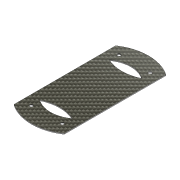
# Autodesk Inventor part: plyta_odbiornik
Saved by Autodesk Inventor 2017 (Build 210142000, 142)
## iProperties
Created: 2017-05-11
Part Number: plyta_odbiornik
Material: Ogólny
Document SubType Name: Modeling
Designer: Kuba01
Density: 1 g/cm^3
Appearance: Domyślna
Author: Kuba01
Autodesk Inventor part; units mm, degrees
ref_plane "YZ Plane" through (0, 0, 0) normal (1, 0, 0) x (0, 1, 0)
ref_plane "XZ Plane" through (0, 0, 0) normal (0, 1, 0) x (-1, 0, 0)
ref_plane "XY Plane" through (0, 0, 0) normal (0, 0, 1) x (1, 0, 0)
sketch "Szkic1" plane through (0, 0, 0) normal (0, 0, 1) x (1, 0, 0)
  circle A0 centre (-19, 53.736463) radius 2
  line L0 (0, -102.826606) -> (0, 109.459635)
  circle A1 centre (51.489502, -156.180896) radius 2
  circle A2 centre (-19, -53.736463) radius 2
  circle A3 centre (19, -53.736463) radius 2
  spline S0 degree 3 poles (-19.948357, 42.291714) (-7.484612, 36.499399) (6.838806, 36.499399) (19.884685, 42.334177) knots -2 -2 -2 -2 -1 -1 -1 -1
  spline S1 degree 3 poles (19.884685, 42.334177) (18.683547, 43.134298) (16.314211, 44.578944) (13.440795, 46.011363) (10.633281, 47.178527) (8.438356, 47.906787) (5.748573, 48.576507) (3.633449, 48.926153) (1.014806, 49.141741) (-1.070138, 49.1397) (-3.689231, 48.918937) (-5.805048, 48.565032) (-8.496008, 47.889736) (-10.692066, 47.156791) (-13.501106, 45.983476) (-16.376096, 44.544624) (-18.746641, 43.094581) (-19.948357, 42.291714) knots -1.92878405 -1.92878405 -1.92878405 -1.92878405 -1.85742515 -1.78606626 -1.75038681 -1.67902792 -1.64334847 -1.57198957 -1.53631013 -1.46495123 -1.42927178 -1.35791289 -1.32223344 -1.25087454 -1.2151951 -1.1438362 -1.0724773 -1.0724773 -1.0724773 -1.0724773
  spline S2 degree 3 poles (-19.948357, -42.291714) (-7.484612, -36.499399) (6.838806, -36.499399) (19.884685, -42.334177) (19.887771, -42.335557) (19.890857, -42.336938) (19.893943, -42.338318) knots -2 -2 -2 -2 -1 -1 -1 -0.99976344 -0.99976344 -0.99976344 -0.99976344
  arc A4 (10.816477, 63.441394) -> (10.816477, 63.441394) centre (0.029646, 15.697095) ccw
  line L1 (-30.717431, -63.122795) -> (-30.717431, 61.299929)
  line L2 (30.776723, 61.29993) -> (30.717431, -63.122795)
  arc A5 (46.460279, 45.179229) -> (46.388819, 45.291469) centre (0.029646, 15.697095) ccw
  arc A6 (30.776723, 61.29993) -> (-30.717431, 61.299929) centre (0.029646, 15.697095) ccw
  arc A7 (-30.717431, -63.122795) -> (30.717431, -63.122795) centre (0, -17.5) ccw
  spline S3 degree 3 poles (19.884685, -42.334177) (18.683547, -43.134298) (16.314211, -44.578944) (13.440795, -46.011363) (10.633281, -47.178527) (8.438356, -47.906787) (5.748573, -48.576507) (3.633449, -48.926153) (1.014806, -49.141741) (-1.070138, -49.1397) (-3.689231, -48.918937) (-5.805048, -48.565032) (-8.496008, -47.889736) (-10.692066, -47.156791) (-13.501106, -45.983476) (-16.376096, -44.544624) (-18.746641, -43.094581) (-19.948357, -42.291714) knots -1.92878405 -1.92878405 -1.92878405 -1.92878405 -1.85742515 -1.78606626 -1.75038681 -1.67902792 -1.64334847 -1.57198957 -1.53631013 -1.46495123 -1.42927178 -1.35791289 -1.32223344 -1.25087454 -1.2151951 -1.1438362 -1.0724773 -1.0724773 -1.0724773 -1.0724773
  arc A8 (-19.985617, 42.471752) -> (20.021799, 42.489012) centre (0, 84.415359) ccw
  arc A9 (20.021799, 42.489012) -> (-19.985617, 42.471752) centre (0.029646, 15.697095) ccw
  arc A10 (31.190436, 27.800736) -> (30.76126, 28.852355) centre (0.029646, 15.697095) ccw
  line L3 (-47.966946, 0) -> (72.77966, 0)
  arc A11 (20.021799, -42.489012) -> (-19.985617, -42.471752) centre (0, -84.415359) ccw
  arc A12 (-19.985617, -42.471752) -> (20.021799, -42.489012) centre (0.029646, -15.697095) ccw
  line L4 (0, -211.709002) -> (0, 162.987741)
  circle A13 centre (19, 53.736463) radius 2
  point P0 (0, 0)
  point P1 (0.029639, 15.697104)
  dimension "d0" = 4
  constraints: 19 point on circle, 14 centre point, 6 end point, 5 symmetric about line, 3 coincident, 2 point on line, 4 other
  measures "d0" diameter of A0
sketch "Szkic1 outline for Wyciągnięcie proste1" plane through (0, 0, 0) normal (0, 0, 1) x (1, 0, 0)
  line L0 (-30.717431, -63.122795) -> (-30.717431, 61.299929)
  arc A0 (30.717431, -63.122795) -> (-30.717431, -63.122795) centre (0, -17.5) cw
  arc A1 (-30.717431, 61.299929) -> (30.776723, 61.29993) centre (0.029646, 15.697095) cw
  line L1 (30.776723, 61.29993) -> (30.717431, -63.122795)
  circle A2 centre (-19, -53.736463) radius 2
  arc A3 (20.021799, -42.489012) -> (-19.985617, -42.471752) centre (0, -84.415359) ccw
  arc A4 (-19.985617, -42.471752) -> (20.021799, -42.489012) centre (0.029646, -15.697095) ccw
  circle A5 centre (19, -53.736463) radius 2
  circle A6 centre (-19, 53.736463) radius 2
  arc A7 (-19.985617, 42.471752) -> (20.021799, 42.489012) centre (0.029646, 15.697095) cw
  arc A8 (20.021799, 42.489012) -> (-19.985617, 42.471752) centre (0, 84.415359) cw
  circle A9 centre (19, 53.736463) radius 2
extrude "Wyciągnięcie proste1" add sketch "Szkic1 outline for Wyciągnięcie proste1" along normal blind 1
sketch "Szkic2" plane through (0, 0, 1) normal (0, 0, 1) x (1, 0, 0)
  spline S0 degree 3 poles (19.066093, -42.869125) (17.919263, -43.604012) (15.656614, -44.931314) (12.910224, -46.24893) (10.224207, -47.323895) (8.121883, -47.995773) (5.542498, -48.61482) (3.51191, -48.938928) (0.996255, -49.139822) (-1.007288, -49.139431) (-3.523026, -48.937545) (-5.553743, -48.612623) (-8.133347, -47.992513) (-10.235885, -47.319744) (-12.922191, -46.24361) (-15.668883, -44.924773) (-17.931768, -43.596446) (-19.078711, -42.861037) knots 1.08873831 1.08873831 1.08873831 1.08873831 1.15730288 1.22586745 1.26014974 1.32871431 1.36299659 1.43156116 1.46584345 1.53440802 1.5686903 1.63725487 1.67153715 1.74010172 1.77438401 1.84294858 1.91151315 1.91151315 1.91151315 1.91151315
  spline S1 degree 2 poles (-19.078711, -42.861037) (-0.031622, -36.330707) (19.066093, -42.869125) knots 1.17954056 1.17954056 1.17954056 1.82085643 1.82085643 1.82085643
  point P0 (0, 0)
extrude "Wyciągnięcie proste2" cut sketch "Szkic2" against normal through all
